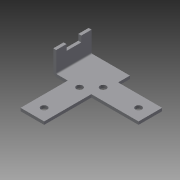
# Autodesk Inventor part: Gusset Connector 2
Saved by Autodesk Inventor 2013 (Build 170138000, 138)
## iProperties
Created: 2013-02-01
Part Number: Gusset Connector 2
Material: Generic
Document SubType Name: Sheet Metal
Designer: actoennies
Density: 1 g/cm^3
Sheet Metal Rule: Default
Author: actoennies
Autodesk Inventor part; units mm, degrees
ref_plane "YZ Plane" through (0, 0, 0) normal (1, 0, 0) x (0, 1, 0)
ref_plane "XZ Plane" through (0, 0, 0) normal (0, 1, 0) x (-1, 0, 0)
ref_plane "XY Plane" through (0, 0, 0) normal (0, 0, 1) x (1, 0, 0)
sketch "Sketch1" plane through (0, 0, 0) normal (0, 1, 0) x (-1, 0, 0)
  circle A0 centre (-63.5, 12.7) radius 3.3782
  circle A1 centre (-25.4, 12.7) radius 3.3782
  circle A2 centre (-12.7, 25.4) radius 3.3782
  circle A3 centre (-12.7, 63.5) radius 3.3782
  line L0 (0, 76.2) -> (0, 25.4)
  line L1 (-25.4, 76.2) -> (0, 76.2)
  line L2 (-25.4, 25.4) -> (-25.4, 76.2)
  line L3 (-76.2, 25.4) -> (-25.4, 25.4)
  line L4 (-76.2, 0) -> (-76.2, 25.4)
  line L5 (-28.829, 0) -> (-76.2, 0)
  line L6 (-9.779, -12.7) -> (15.621, -12.7)
  line L7 (15.621, -12.7) -> (15.621, 25.4)
  line L8 (15.621, 25.4) -> (0, 25.4)
  line L9 (15.621, -12.7) -> (-28.829, -12.7)
  line L10 (-28.829, -12.7) -> (-28.829, 0)
  point P0 (0, 0)
  point P1 (0, 0)
  dimension "d0" = 44.45
  measures "d0" distance of L6.end L9.end
extrude "Plate1" add sketch "Sketch1" along normal blind 3.175
sketch "Sketch2" plane through (-12.446, 0, 25.4) normal (-1, 0, 0) x (0, -1, 0)
  line L0 (0, -38.1) -> (0, 0)
  line L1 (0, 0) -> (-25.4, 0)
  line L2 (-25.4, 0) -> (-25.4, -38.1)
  line L3 (-25.4, -38.1) -> (0, -38.1)
  constraints: 6 end point, 1 horizontal, 1 perpendicular, 1 vertical
edge flange "Flange1" height 25.4 angle 90 thickness 3.175 bend radius 1.27 thickness toward (-1, 0, 0) relief straight relief width 3.175 relief depth 1.5875 edges at (-15.621, 3.175, 6.35) wall of the first edge with corners at (-12.446, 0, -12.7) (-12.446, 0, 25.4) (-12.446, 25.4, 25.4) (-12.446, 25.4, -12.7)
bend "Bend1"
corner "Corner1"
sketch "Sketch3" plane through (-12.446, 25.4, 25.4) normal (1, 0, 0) x (0, 0, -1)
  line L0 (38.1, 0) -> (38.1, -20.955) projected
  line L1 (38.1, 0) -> (0, 0) projected
  line L2 (0, 0) -> (0, -20.955) projected
  line L3 (11.1125, 0) -> (11.1125, -6.35)
  line L4 (11.1125, -6.35) -> (26.9875, -6.35)
  line L5 (26.9875, -6.35) -> (26.9875, 0)
  point P0 (25.4, -25.4)
  dimension "d12" = 6.35
  dimension "d13" = 15.875
  dimension "d14" = 11.1125
  constraints: 6 end point, 2 perpendicular, 2 point on line, 1 parallel
  measures "d12" distance of L3.start L3.end
  measures "d13" distance of L3.end L4.end
  measures "d14" distance between parallel lines of L0 L5
extrude "Cut1" cut sketch "Sketch3" against normal blind 3.175
equation "\"d15\" = Thickness"
equation "\"d2\" = BendReliefWidth"
equation "\"d3\" = BendReliefDepth"
equation "\"d4\" = MinimumRemnant"
equation "\"d5\" = BendRadius"
equation "\"d9\" = CornerReliefSize"
equation "\"d10\" = GapSize"
equation "\"d11\" = JacobiRadiusSize"
equation "\"BendRadius\" = Thickness"
equation "\"BendReliefWidth\" = Thickness"
equation "\"BendReliefDepth\" = 0.5 * Thickness"
equation "\"CornerReliefSize\" = 4 * Thickness"
equation "\"MinimumRemnant\" = 2 * Thickness"
equation "\"TransitionRadius\" = BendRadius"
equation "\"JacobiRadiusSize\" = BendRadius"
equation "\"GapSize\" = Thickness"
equation "\"d1\" = BendRadius"
equation "\"Thickness\" = 3.175"
body "Solid1"
